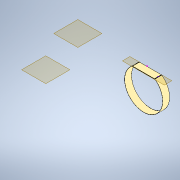
# Autodesk Inventor part: Small_Ring
Saved by Autodesk Inventor 2021 (Build 250183000, 183)
## iProperties
Created: 2020-05-27
Part Number: Small_Ring
Material: Iron, Cast
Document SubType Name: Modeling
Designer: aydan
Density: 7.15 g/cm^3
Appearance: Gold - Metal
Author: aydan
Autodesk Inventor part; units mm, degrees
ref_plane "YZ Plane" through (0, 0, 0) normal (1, 0, 0) x (0, 1, 0)
ref_plane "XY Plane" through (0, 0, 0) normal (0, 0, 1) x (1, 0, 0)
sketch "Sketch3" plane through (0, 0, 0) normal (0, 0, 1) x (1, 0, 0)
  circle A0 centre (0, 0) radius 17.25
  circle A1 centre (0, 0) radius 17.375
  dimension "d8" = 34.5
  dimension "d9" = 34.75
  constraints: 2 centre point, 2 coincident
  measures "d8" diameter of A0
  measures "d9" diameter of A1
extrude "Extrusion3" add sketch "Sketch3" along normal mid plane 6.25
sketch "Sketch4" plane through (0, 0, 3.125) normal (0, 0, 1) x (1, 0, 0)
  circle A0 centre (0, 0) radius 17.375
  circle A1 centre (0, 0) radius 17.625
  dimension "d12" = 34.75
  dimension "d13" = 0.25
  constraints: 2 centre point, 1 coincident
  measures "d12" diameter of A0
  measures "d13" radial gap between concentric circles of A0 A1
extrude "Extrusion4" cut sketch "Sketch4" along normal blind 0.25 and the other way blind 5.75
ref_plane "Work Plane4" through (0, 17.5, 0) normal (0, 1, 0) x (-1, 0, 0)
sketch "Sketch6" plane through (0, 17.5, 0) normal (0, 1, 0) x (-1, 0, 0)
  line L0 (-10, 3.75) -> (10, 3.75)
  line L1 (10, 3.75) -> (10, -3.75)
  line L2 (10, -3.75) -> (-10, -3.75)
  line L3 (-10, -3.75) -> (-10, 3.75)
  line L4 (-10, 3.75) -> (10, -3.75) construction
  line L5 (10, 3.75) -> (-10, -3.75) construction
  point P0 (0, 0)
  dimension "d19" = 20
  dimension "d20" = 7.5
  constraints: 12 end point, 2 midpoint, 2 parallel, 1 horizontal, 1 perpendicular
  measures "d19" distance of L1.end L2.end
  measures "d20" distance between parallel lines of L2 L0
extrude "Extrusion5" cut sketch "Sketch6" against normal blind 10
ref_plane "Work Plane3" through (0, 17.5, 0) normal (0, 1, 0) x (-1, 0, 0)
sketch "Sketch7" plane through (0, 17.5, 0) normal (0, 1, 0) x (-1, 0, 0)
  point P0 (0, 0)
sketch "Sketch8" plane through (10, 14.0557, -3.125) normal (-1, 0, 0) x (0, 0, 1)
  line L0 (6.25, 0) -> (0, 0)
  line L1 (0, 0) -> (0, 0.1531)
  line L2 (0, 0.1531) -> (6.25, 0.1531)
  line L3 (6.25, 0.1531) -> (0, 0.1531) projected
  point P0 (3.125, 0.1531)
  point P1 (3.125, 0.1531)
  constraints: 6 end point, 2 midpoint, 1 coincident, 1 parallel, 1 perpendicular
ref_plane "Work Plane5" through (0, 13.8, 0) normal (0, 1, 0) x (-1, 0, 0)
sketch "Sketch9" plane through (0, 13.8, 0) normal (0, 1, 0) x (-1, 0, 0)
  line L0 (-10, -3.125) -> (-10, 3.125) projected
  line L1 (10, -3.125) -> (-10, -3.125)
  line L2 (-10, -3.125) -> (-10, 3.125)
  line L3 (-10, 3.125) -> (10, 3.125)
  line L4 (10, 3.125) -> (10, -3.125)
  point P0 (0, 0)
  constraints: 8 end point, 2 parallel, 1 horizontal, 1 perpendicular
extrude "Extrusion6" add sketch "Sketch9" along normal blind 0.25
body "Solid2"
